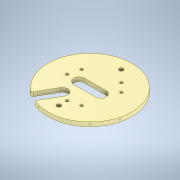
# Autodesk Inventor part: End Cap
Saved by Autodesk Inventor 2021 (Build 250183000, 183)
## iProperties
Created: 2020-11-18
Part Number: End Cap
Material: Generic
Document SubType Name: Modeling
Designer: dsouthall
Density: 1 g/cm^3
Appearance: Nylon 6
Author: dsouthall
Autodesk Inventor part; units mm, degrees
ref_plane "YZ Plane" through (0, 0, 0) normal (1, 0, 0) x (0, 1, 0)
ref_plane "XZ Plane" through (0, 0, 0) normal (0, 1, 0) x (-1, 0, 0)
ref_plane "XY Plane" through (0, 0, 0) normal (0, 0, 1) x (1, 0, 0)
sketch "Cylinders Sketch" plane through (0, 0, 0) normal (0, 1, 0) x (-1, 0, 0)
  arc A0 (34.3178, 92.2484) -> (62.7306, 75.8443) centre (0, 0) ccw
  line L0 (35.9604, 87.6852) -> (12.6464, 47.3042)
  line L1 (57.9574, 74.9852) -> (34.6435, 34.6042)
  line L2 (187.4055, 0) -> (-188.0938, 0) projected
  line L3 (49.2125, 85.2386) -> (23.6449, 40.9542) construction
  arc A1 (34.6435, 34.6042) -> (12.6464, 47.3042) centre (23.6449, 40.9542) ccw construction
  line L4 (34.6435, 34.6042) -> (26.7764, 20.9781) construction
  line L5 (12.6464, 47.3042) -> (4.7794, 33.6781) construction
  arc A2 (12.6464, 47.3042) -> (34.6435, 34.6042) centre (23.6449, 40.9542) ccw
  arc A3 (49.2125, 85.2386) -> (37.8026, 90.876) centre (0, 0) ccw construction
  arc A4 (59.7996, 78.176) -> (49.2125, 85.2386) centre (0, 0) ccw construction
  line L6 (0, -187.993) -> (0, 186.8008) projected
  line L7 (25.4, 0) -> (-11.3539, 0) construction
  arc A5 (25.4, -12.7) -> (25.4, 12.7) centre (25.4, 0) ccw
  arc A6 (-25.4, 12.7) -> (-25.4, -12.7) centre (-25.4, 0) ccw
  line L8 (25.4, 12.7) -> (-25.4, 12.7)
  line L9 (-25.4, -12.7) -> (25.4, -12.7)
  arc A7 (25.4, 12.7) -> (25.4, -12.7) centre (25.4, 0) ccw construction
  arc A8 (-25.4, -12.7) -> (-25.4, 12.7) centre (-25.4, 0) ccw construction
  arc A9 (62.7306, 75.8443) -> (57.9574, 74.9852) centre (60.707, 73.3977) ccw
  arc A10 (35.9604, 87.6852) -> (34.3178, 92.2484) centre (33.2107, 89.2727) ccw
  dimension "d0" = 0
  dimension "d1" = 0
  dimension "d5" = 25.4
  dimension "d6" = 60
  dimension "d7" = 12.7
  dimension "d9" = 25.4
  dimension "d12" = 98.425
  dimension "d13" = 51.1351
  dimension "d14" = 60
  dimension "d15" = 25.4
  dimension "d16" = 0
  dimension "d17" = 0
  dimension "d25" = 0
  dimension "d31" = 12.7
  dimension "d32" = 50.8
  dimension "d33" = 0
  dimension "d34" = 12.7
  dimension "d35" = 25.4
  dimension "d81" = 3.175
  constraints: 24 point on circle, 16 end point, 11 centre point, 7 tangent, 4 parallel, 2 equal radius, 2 line through centre, 2 point on line
  measures "d0" distance of point (0, 0) A0.centre
  measures "d1" distance of point (0, 0) A0.centre
  measures "d5" distance between parallel lines of L0 L1
  measures "d6" angle of L1 L2
  measures "d7" distance from line of point (0, 0) L1
  measures "d9" distance of L4.end L5.end
  measures "d12" distance of A0.centre L3.start
  measures "d13" distance of L3.start L3.end
  measures "d14" angle of L3 L2
  measures "d15" diameter of A1
  measures "d16" distance of A1.centre L3.end
  measures "d17" distance of A1.centre L3.end
  measures "d25" distance from line of L2 L7.end
  measures "d31" radius of A5
  measures "d32" distance of A6.centre A5.centre
  measures "d33" vertical distance of A6.centre A5.centre
  measures "d34" distance between parallel lines of L2 L8
  measures "d35" distance from line of A6.centre L6
  measures "d81" radius of A9
extrude "Cylinders Cutout" add sketch "Cylinders Sketch" along normal blind 9.652 contours A10 L0 A2 L1 A9 A0 L2 A5 L8 L6 | L6 L8 A6 L2 A0 | L2 A6 L9 L6 A0 | L6 L9 A5 L2 A0
sketch "Wedges Sketch" plane through (0, 9.652, 0) normal (0, 1, 0) x (1, 0, 0)
  line L0 (0, 0) -> (-66.1046, 8.7028) construction
  arc A0 (-34.3178, -92.2484) -> (-62.7306, -75.8443) centre (0, 0) ccw construction
  line L1 (-57306.7077, 0) -> (57306.2964, 0) construction
  line L2 (0, 0) -> (-40.5892, 52.8968) construction
  arc A1 (-91.2873, 12.0182) -> (-91.2873, -12.0182) centre (0, 0) ccw construction
  arc A2 (-66.1046, 8.7028) -> (-66.1046, -8.7028) centre (0, 0) ccw construction
  arc A3 (-58.6248, 70.9996) -> (-90.7998, 15.2708) centre (0, 0) ccw
  arc A4 (-42.9516, 50.9972) -> (-65.6407, 11.6986) centre (0, 0) ccw
  line L3 (-56.0517, 73.048) -> (-59.9173, 78.0858) construction
  line L4 (-42.478, 55.3585) -> (-54.0844, 70.4841)
  line L5 (-91.2873, 12.0182) -> (-97.583, 12.847) construction
  line L6 (-69.1808, 9.1078) -> (-88.0832, 11.5964)
  line L7 (-60.4672, -64.0922) -> (-50.4876, -46.8071)
  line L8 (-57.9574, -74.9852) -> (-34.6435, -34.6042) construction
  line L9 (0, 0) -> (-66.1046, -8.7028) construction
  arc A5 (-90.7998, -15.2708) -> (-65.4746, -64.7371) centre (0, 0) ccw
  arc A6 (65.6407, 11.6986) -> (-40.5892, 52.8968) centre (0, 0) ccw construction
  arc A7 (-65.6407, -11.6986) -> (-50.8174, -43.1642) centre (0, 0) ccw
  arc A8 (90.7998, 15.2708) -> (58.6248, 70.9996) centre (0, 0) ccw construction
  line L10 (-69.1808, -9.1078) -> (-88.0832, -11.5964)
  line L11 (0, 0) -> (0, 124.9031) construction
  line L12 (57306.7077, 0) -> (-57306.2964, 0) construction
  arc A9 (90.7998, 15.2708) -> (56.0517, 73.048) centre (0, 0) ccw
  arc A10 (65.6407, 11.6986) -> (42.9516, 50.9972) centre (0, 0) ccw
  line L13 (42.478, 55.3585) -> (54.0844, 70.4841)
  line L14 (69.1808, 9.1078) -> (88.0832, 11.5964)
  arc A11 (58.6248, -70.9996) -> (90.7998, -15.2708) centre (0, 0) ccw
  line L15 (69.1808, -9.1078) -> (88.0832, -11.5964)
  arc A12 (42.9516, -50.9972) -> (65.6407, -11.6986) centre (0, 0) ccw
  line L16 (42.478, -55.3585) -> (54.0844, -70.4841)
  arc A13 (-65.4746, -64.7371) -> (-60.4672, -64.0922) centre (-63.2168, -62.5047) ccw
  arc A14 (-50.4876, -46.8071) -> (-50.8174, -43.1642) centre (-53.2373, -45.2196) ccw
  arc A15 (-65.6407, -11.6986) -> (-69.1808, -9.1078) centre (-68.7664, -12.2557) ccw
  arc A16 (-88.0832, -11.5964) -> (-90.7998, -15.2708) centre (-87.6688, -14.7442) ccw
  arc A17 (-90.7998, 15.2708) -> (-88.0832, 11.5964) centre (-87.6688, 14.7442) ccw
  arc A18 (-54.0844, 70.4841) -> (-58.6248, 70.9996) centre (-56.6033, 68.5513) ccw
  arc A19 (-42.9516, 50.9972) -> (-42.478, 55.3585) centre (-44.9969, 53.4256) ccw
  arc A20 (42.478, 55.3585) -> (42.9516, 50.9972) centre (44.9969, 53.4256) ccw
  arc A21 (-69.1808, 9.1078) -> (-65.6407, 11.6986) centre (-68.7664, 12.2557) ccw
  arc A22 (58.6248, 70.9996) -> (54.0844, 70.4841) centre (56.6033, 68.5513) ccw
  arc A23 (65.6407, 11.6986) -> (69.1808, 9.1078) centre (68.7664, 12.2557) ccw
  arc A24 (65.6407, 11.6986) -> (69.1808, 9.1078) centre (68.7664, 12.2557) ccw
  arc A25 (88.0832, 11.5964) -> (90.7998, 15.2708) centre (87.6688, 14.7442) ccw
  arc A26 (88.0832, 11.5964) -> (90.7998, 15.2708) centre (87.6688, 14.7442) ccw
  arc A27 (90.7998, -15.2708) -> (88.0832, -11.5964) centre (87.6688, -14.7442) ccw
  arc A28 (69.1808, -9.1078) -> (65.6407, -11.6986) centre (68.7664, -12.2557) ccw
  arc A29 (42.9516, -50.9972) -> (42.478, -55.3585) centre (44.9969, -53.4256) ccw
  arc A30 (54.0844, -70.4841) -> (58.6248, -70.9996) centre (56.6033, -68.5513) ccw
  point P0 (-37.8026, -90.876)
  point P1 (-59.7996, -78.176)
  point P2 (91.2873, 12.0182)
  point P3 (40.5892, 52.8968)
  point P4 (66.1046, 8.7028)
  point P5 (56.0517, -73.048)
  point P6 (91.2873, -12.0182)
  point P7 (66.1046, -8.7028)
  point P8 (40.5892, -52.8968)
  point P9 (58.6248, 70.9996)
  dimension "d38" = 7.5
  dimension "d39" = 45
  dimension "d41" = 25.4
  dimension "d42" = 6.35
  dimension "d43" = 7.5
  dimension "d44" = 45
  dimension "d45" = 7.5
  dimension "d46" = 7.62
  dimension "d47" = 7.5
  dimension "d50" = 3.175
  constraints: 75 point on circle, 36 tangent, 30 centre point, 30 end point, 17 equal radius, 16 point on line, 10 symmetric about line, 2 concentric, 1 parallel, 1 vertical, 4 other
  measures "d38" angle of L1 L0
  measures "d39" angle of L0 L2
  measures "d41" radial gap between concentric circles of A1 A2
  measures "d42" radial gap between concentric circles of A0 A1
  measures "d43" angle of L1 L6
  measures "d44" angle of L6 L4
  measures "d45" angle of L1 L9
  measures "d46" distance between parallel lines of L8 L7
  measures "d47" angle of L1 L10
  measures "d50" radius of A13
extrude "Wedges Cutout" [suppressed]
sketch "Rope Holes Sketch" plane through (0, 9.652, 0) normal (0, 1, 0) x (1, 0, 0)
  circle A0 centre (0, 0) radius 38.1 construction
  arc A1 (-34.3178, -92.2484) -> (-62.7306, -75.8443) centre (0, 0) ccw projected
  line L0 (19.05, -32.9956) -> (-19.05, 32.9956) construction
  line L1 (-187.4055, 0) -> (188.0938, 0) construction
  circle A2 centre (-19.05, 32.9956) radius 4.7625 construction
  circle A3 centre (19.05, -32.9956) radius 4.7625 construction
  circle A4 centre (0, -73.025) radius 4.7625
  circle A5 centre (0, 73.025) radius 4.7625
  line L2 (0, 187.993) -> (0, -186.8008) construction
  point P0 (-37.8026, -90.876)
  point P1 (-59.7996, -78.176)
  dimension "d51" = 38.1
  dimension "d52" = 60
  dimension "d53" = 0
  dimension "d54" = 0
  dimension "d55" = 0
  dimension "d56" = 0
  dimension "d57" = 9.525
  dimension "d58" = 0
  dimension "d59" = 146.05
  dimension "d60" = 0
  dimension "d61" = 73.025
  constraints: 5 centre point, 3 equal radius, 2 end point, 2 point on circle, 1 concentric, 1 line through centre
  measures "d51" radius of A0
  measures "d52" angle of L1 L0
  measures "d53" distance of L0.end A2.centre
  measures "d54" distance of L0.end A2.centre
  measures "d55" distance of A3.centre L0.start
  measures "d56" distance of L0.start A3.centre
  measures "d57" diameter of A2
  measures "d58" horizontal distance of A5.centre A4.centre
  measures "d59" distance of A5.centre A4.centre
  measures "d60" distance from line of L2 A5.centre
  measures "d61" distance of point (0, 0) A5.centre
extrude "Rope Holes Cutout" cut sketch "Rope Holes Sketch" against normal blind 24.13
sketch "Support Holes Sketch" plane through (0, 9.652, 0) normal (0, 1, 0) x (1, 0, 0)
  circle A0 centre (0, 0) radius 53.6399 construction
  arc A1 (-34.3178, -92.2484) -> (-62.7306, -75.8443) centre (0, 0) ccw projected
  circle A2 centre (-53.6399, 0) radius 3.175
  line L0 (-187.4055, 0) -> (188.0938, 0) projected
  line L1 (0, 187.993) -> (0, -186.8008) construction
  circle A3 centre (26.8199, -46.4535) radius 3.175
  circle A4 centre (26.8199, 46.4535) radius 3.175
  circle A5 centre (0, -53.6399) radius 3.175
  circle A6 centre (46.4535, 26.8199) radius 3.175
  circle A7 centre (-46.4535, 26.8199) radius 3.175
  point P0 (-37.8026, -90.876)
  point P1 (-59.7996, -78.176)
  dimension "d64" = 53.6399
  dimension "d66" = 0
  dimension "d67" = 53.6399
  dimension "d68" = 6.35
  dimension "d71" = 360
  dimension "d73" = 0
  dimension "d74" = 53.6399
  dimension "d77" = 360
  constraints: 7 centre point, 1 concentric, 1 equal radius, 14 other
  measures "d64" radius of A0
  measures "d66" distance from line of L0 A2.centre
  measures "d67" distance from line of L1 A2.centre
  measures "d68" diameter of A2
  measures "d73" distance from line of L1 A5.centre
  measures "d74" distance from line of L0 A5.centre
extrude "Support Holes Cutout" cut sketch "Support Holes Sketch" against normal blind 24.13 contours L0 A2 | A2 L0 | A3 | A4 | A5 | A6 | A7
sketch "Set Screw Sketch" plane through (0, 9.652, 0) normal (0, 1, 0) x (1, 0, 0)
  line L0 (-122.6726, -32.87) -> (122.6726, 32.87) construction
  line L1 (-32.87, 122.6726) -> (32.87, -122.6726) construction
  line L2 (-187.4055, 0) -> (188.0938, 0) construction
  line L3 (0, 187.993) -> (0, -186.8008) projected
  arc A0 (-34.3178, -92.2484) -> (-62.7306, -75.8443) centre (0, 0) ccw projected
  line L4 (69.597, -69.597) -> (-69.597, 69.597) construction
  line L5 (-25.4743, -95.0712) -> (25.4743, 95.0712) construction
  line L6 (-95.0712, 25.4743) -> (95.0712, -25.4743) construction
  line L7 (-69.597, -69.597) -> (69.597, 69.597) construction
  dimension "d82" = 254
  dimension "d83" = 0
  dimension "d84" = 0
  dimension "d85" = 127
  dimension "d86" = 127
  dimension "d89" = 15
  dimension "d93" = 30
  dimension "d94" = 30
  dimension "d95" = 30
  dimension "d96" = 30
  constraints: 12 end point, 2 coincident, 2 perpendicular, 13 other
  measures "d82" distance of L0.start L0.end
  measures "d83" distance from line of L0 point (0, 0)
  measures "d84" distance from line of point (0, 0) L1
  measures "d85" distance of point (0, 0) L0.start
  measures "d86" distance of point (0, 0) L1.start
  measures "d89" angle of L3 L1
  measures "d93" angle of L1 L4
  measures "d94" angle of L1 L5
  measures "d95" angle of L7 L0
  measures "d96" angle of L0 L6
ref_plane "Edge Hole Plane 1" through (69.597, 9.652, 69.597) normal (0.7071068, 0, 0.7071068) x (0, 1, 0)
ref_plane "Edge Hole Plane 2" through (-25.4743, 9.652, 95.0712) normal (-0.258819, 0, 0.9659258) x (0, -1, 0)
sketch "Edge Hole Center 1" plane through (69.597, 9.652, 69.597) normal (0.7071068, 0, 0.7071068) x (0, 1, 0)
  line L0 (0, -98.425) -> (0, 98.425) projected
  point P0 (-9.652, 0)
  point P1 (-4.826, 0)
  point P2 (0, 89.4958)
  point P3 (0, 97.9872)
  dimension "d97" = 4.826
  dimension "d98" = 0
  measures "d97" distance from line of L0 point (-4.826, 0)
  measures "d98" vertical distance of point (-9.652, 0) point (-4.826, 0)
sketch "Edge Hole Center 2" plane through (-25.4743, 9.652, 95.0712) normal (-0.258819, 0, 0.9659258) x (0, -1, 0)
  line L0 (0, 98.425) -> (0, -98.425) projected
  line L1 (9.652, 98.425) -> (9.652, -98.425) projected
  point P0 (9.652, 0)
  point P1 (4.826, 0)
  point P2 (0, -9.2728)
  point P3 (0, -40.9632)
  point P4 (9.652, -9.2728)
  point P5 (9.652, -40.9632)
  dimension "d100" = 0
  dimension "d167" = 4.826
  measures "d100" vertical distance of point (9.652, 0) point (4.826, 0)
  measures "d167" distance from line of point (4.826, 0) L1
ref_plane "Central Plane" through (0, 4.826, 0) normal (0, 1, 0) x (1, 0, 0)
hole "Insert Edge Hole 1" [suppressed]
hole "Insert Edge Hole 2" [suppressed]
pattern_circular "Circular Pattern2" [suppressed]
hole "4-40 2" at (-25.4743, 4.826, 95.0712) direction (0.258819, 0, -0.9659258) diameter 2.1565 depth 8.8646 tip angle 118 thread size "4-40 UNC" class "2B" standard "ANSI Unified Screw Threads"
hole "4-40 1" at (69.597, 4.826, 69.597) direction (-0.7071068, 0, -0.7071068) diameter 2.1565 depth 8.8646 tip angle 118 thread size "4-40 UNC" class "2B" standard "ANSI Unified Screw Threads"
pattern_circular "Circular Pattern3" count 4 over 360 about axis through (0, -10, 0) along (0, 1, 0) of "4-40 2", "4-40 1"
equation "\"d7\" = 0.5 * d5"
equation "\"d12\" = 0.5 * d3"
equation "\"d3\" = 196.85"
body "Solid1"
